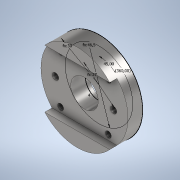
# Autodesk Inventor part: Flansch_FemalePart_MainAxis_HeadConnectorBase_V2
Saved by Autodesk Inventor 2022 (Build 260153000, 153)
## iProperties
Created: 2022-07-15
Part Number: Flansch_FemalePart_MainAxis_HeadConnectorBase_V2
Material: Edelstahl
Document SubType Name: Modeling
Designer: alexw
Density: 8 g/cm^3
Appearance: Halbpoliert
Mass: 1053.61 g
Surface Area: 257.092 cm^2
Volume: 131.701 cm^3
Flansch_ParralelMech_FlatPart_Width: 140,000 mm
Total_Bearing_Hole_Dist: 80,000 mm
MainAxis_Schluesselweite: 24,000 mm
Author: alexw
Autodesk Inventor part; units mm, degrees
ref_plane "YZ Plane" through (0, 0, 0) normal (1, 0, 0) x (0, 1, 0)
ref_plane "XZ Plane" through (0, 0, 0) normal (0, 1, 0) x (-1, 0, 0)
ref_plane "XY Plane" through (0, 0, 0) normal (0, 0, 1) x (1, 0, 0)
sketch "Skizze1" plane through (0, 0, 0) normal (0, 0, 1) x (1, 0, 0)
  circle A0 centre (0, 0) radius 30
  circle A1 centre (0, 0) radius 13.5
  circle A2 centre (0, 0) radius 9.5
  circle A3 centre (0, 0) radius 23.25 construction
  line L0 (0, 0) -> (16.4402, 16.4402) construction
  line L1 (0, 0) -> (0, 30) construction
  point P0 (-16.4402, 16.4402)
  point P1 (-16.4402, -16.4402)
  point P2 (16.4402, -16.4402)
  dimension "d3" = 30
  dimension "d4" = 46.5
  dimension "d0" = 4
  dimension "d1" = 27
  dimension "d7" = 360
  dimension "d99" = 45
  constraints: 4 coincident, 4 end point, 2 centre point, 1 vertical, 1 vertical alignment, 10 other
  measures "d0" radial gap between concentric circles of A2 A1
  measures "d1" diameter of A1
  measures "d99" angle of L1 L0
extrude "Extrusion1" add sketch "Skizze1" along normal blind 15 contours A0 | A1
extrude "Extrusion2" add sketch "Skizze1" against normal blind 2.6 contours A1
sketch "Skizze2" plane through (0, 0, 15) normal (0, 0, 1) x (1, 0, 0)
  point P0 (0, 0)
  point P1 (16.4402, 16.4402)
  point P2 (16.4402, -16.4402)
  point P3 (-16.4402, -16.4402)
  point P4 (-16.4402, 16.4402)
hole "Bohrung1" at (16.4402, 16.4402, 15) at (16.4402, -16.4402, 15) at (-16.4402, -16.4402, 15) at (-16.4402, 16.4402, 15) direction (0, 0, -1) diameter 4.134 end through all thread size "M5x0.8" class "6H" standard "ISO Metric profile"
ref_plane "Arbeitsebene1" through (0, 0, 10) normal (0, 0, 1) x (1, 0, 0)
sketch "Skizze10" plane through (0, 0, 15) normal (0, 0, 1) x (1, 0, 0)
  line L0 (-30, 20) -> (30, 20)
  line L1 (30, 20) -> (30, -20)
  line L2 (30, -20) -> (-30, -20)
  line L3 (-30, -20) -> (-30, 20)
  line L4 (-30, 20) -> (30, -20) construction
  line L5 (30, 20) -> (-30, -20) construction
  circle A0 centre (0, 0) radius 30 projected
  circle A1 centre (-16.4402, 16.4402) radius 2.067 construction
  circle A2 centre (-16.4402, -16.4402) radius 2.067 construction
  line L6 (-20, 0) -> (20, 0) construction
  circle A3 centre (0, 0) radius 30 projected
  line L7 (0, 42) -> (0, -42) construction
  point P0 (-22.3607, 20)
  point P1 (-22.3607, -20)
  point P2 (22.3607, -20)
  point P3 (22.3607, 20)
  point P4 (30, 0)
  point P5 (-30, 0)
  dimension "d81" = 40
  dimension "d82" = 40
  constraints: 14 end point, 4 midpoint, 2 horizontal, 2 parallel, 1 perpendicular, 1 tangent
  measures "d81" distance between parallel lines of L0 L2
  measures "d82" distance of L6.end L6.start
extrude "Extrusion7" cut sketch "Skizze10" against normal blind 5 contours L0 A0 L3 | L0 A0 L2 | A0 L2 L3 | L0 L1 A0 | L1 L2 A0
sketch "Skizze11" plane through (0, 0, 0) normal (0, 0, -1) x (-1, 0, 0)
  point P0 (0, 0)
  point P1 (-20, 0)
  point P2 (20, 0)
hole "Bohrung4" at (20, 0, 0) at (-20, 0, 0) direction (0, 0, 1) diameter 4.5 end through all countersink diameter 9.4 countersink angle 90 clearance for "Senkschraube mit Linsenkopf ISO 2010" size "M4" standard "DIN"
sketch "Skizze4" plane through (0, 0, 0) normal (1, 0, 0) x (0, 1, 0)
  line L0 (9.5, -2.6) -> (-9.5, -2.6) construction
  line L1 (0, 192.52) -> (0, -35.12) construction
  line L2 (-9.5, 15) -> (-9.5, -2.6) construction
  line L3 (9.5, 15) -> (9.5, -2.6) construction
  line L4 (-9.5, 15) -> (9.5, 15) construction
  line L5 (-9.5, 2.4) -> (9.5, 2.4)
  line L6 (-9.5, 2.4) -> (-9.5, 15)
  line L7 (-9.5, 15) -> (-20, 15)
  line L8 (-20, 15) -> (-20, 165)
  line L9 (-20, 165) -> (20, 165)
  line L10 (20, 15) -> (9.5, 15)
  line L11 (9.5, 15) -> (9.5, 2.4)
  line L12 (20, 165) -> (20, 15)
  line L13 (0, 2.4) -> (0, 165)
  point P0 (0, 0)
  dimension "d27" = 5
  dimension "d31" = 150
  dimension "d33" = 40
  dimension "MainAxis_Schluesselweite" = 24
  dimension "d46" = 1
  dimension "d52" = 32
  dimension "Flansch_ParralelMech_FlatPart_Width" = 140
  constraints: 6 end point, 6 point on circle, 2 concentric, 2 vertical, 1 centre point, 1 horizontal, 1 parallel
  measures "Flansch_ParralelMech_FlatPart_Width" distance between parallel lines of L0 L1
sketch "Skizze7" plane through (0, 0, 50) normal (0, 0, 1) x (1, 0, 0)
  line L0 (-12, 16) -> (-12, -16) construction
  line L1 (-12, 15) -> (-3, 15)
  line L2 (-3, 15) -> (-3, 11.425)
  line L3 (-3, 11.425) -> (3, 11.425)
  line L4 (3, 11.425) -> (3, 15)
  line L5 (3, 15) -> (12, 15)
  line L6 (-12, 0) -> (-12, 15)
  line L7 (0, -16) -> (0, 16) construction
  line L8 (12, -16) -> (12, 16) construction
  line L9 (12, 15) -> (12, 0)
  line L10 (-12, 0) -> (12, 0)
  line L11 (-42, 0) -> (42, 0) construction
  point P0 (0, 11.425)
  point P1 (-12, -7.2111)
  point P2 (12, 7.2111)
  dimension "d51" = 9
  dimension "d63" = 30
  dimension "d64" = 22.85
  constraints: 16 end point, 5 point on line, 4 perpendicular, 3 midpoint, 1 horizontal, 1 vertical
  measures "d51" distance between parallel lines of L0 L2
  measures "d63" diameter of L1 L10
  measures "d64" diameter of L3 L10
sketch "Skizze8" plane through (12, -16, 160) normal (1, 0, 0) x (0, 0, -1)
  line L0 (30, -26) -> (30, 58) construction
  line L1 (-32.52, 16) -> (195.12, 16) construction
  point P0 (160, 16)
  point P1 (30, 16)
  constraints: 1 midpoint, 1 point on line
equation "\"d3\" = Flansch_FemalePart_OuterDia"
equation "\"d4\" = Flansch_FemalePart_HoleDia"
equation "\"d1\" = Flansch_Klemmdeckelausnahme_Dia"
equation "\"d33\" = d28"
equation "\"Total_Bearing_Hole_Dist\" = 80"
equation "\"Flansch_FemalePart_OuterDia\" = 30"
equation "\"Flansch_FemalePart_HoleDia\" = 46.5"
equation "\"Flansch_Klemmdeckelausnahme_Dia\" = 27"
equation "\"d28\" = 40"
